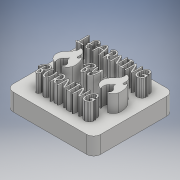
# Autodesk Inventor part: LearningByBurning
Saved by Autodesk Inventor 2017 (Build 210142000, 142)
## iProperties
Created: 2019-02-26
Part Number: LearningByBurning
Material: Generic
Document SubType Name: Modeling
Designer: Daniel Serena
Density: 1 g/cm^3
Appearance: Default
Author: Daniel Serena
Autodesk Inventor part; units mm, degrees
(part 1 of 2)
ref_plane "YZ Plane" through (0, 0, 0) normal (1, 0, 0) x (0, 1, 0)
ref_plane "XZ Plane" through (0, 0, 0) normal (0, 1, 0) x (-1, 0, 0)
ref_plane "XY Plane" through (0, 0, 0) normal (0, 0, 1) x (1, 0, 0)
sketch "Sketch1" plane through (0, 0, 0) normal (0, 0, 1) x (1, 0, 0)
  line L0 (-10.4772, 8.2772) -> (11.5644, 8.2772) construction
  line L1 (11.5644, 8.2772) -> (11.5644, -9.0375) construction
  line L2 (11.5644, -9.0375) -> (-10.4772, -9.0375) construction
  line L3 (-10.4772, -9.0375) -> (-10.4772, 8.2772) construction
  line L4 (-8.5891, 8.1961) -> (-8.5771, 8.1961)
  spline S0 degree 2 poles (-8.5771, 8.1961) (-8.4601, 8.1961) (-8.403, 8.0731) knots 0 0 0 1 1 1
  spline S1 degree 2 poles (-8.403, 8.0731) (-8.379, 8.0341) (-8.361, 7.6799) knots 0 0 0 1 1 1
  spline S2 degree 2 poles (-8.361, 7.6799) (-8.328, 7.0105) (-8.328, 6.3291) knots 0 0 0 1 1 1
  spline S3 degree 2 poles (-8.328, 6.3291) (-8.328, 5.4976) (-8.382, 5.0654) knots 0 0 0 1 1 1
  line L5 (-8.382, 5.0654) -> (-8.379, 5.0654)
  spline S4 degree 2 poles (-8.379, 5.0654) (-7.9408, 5.1764) (-7.6826, 5.1764) knots 0 0 0 1 1 1
  line L6 (-7.6826, 5.1764) -> (-7.6766, 5.1764)
  spline S5 degree 2 poles (-7.6766, 5.1764) (-7.3314, 5.1764) (-7.0733, 5.0143) knots 0 0 0 1 1 1
  spline S6 degree 2 poles (-7.0733, 5.0143) (-7.0072, 4.9483) (-7.0072, 4.8672) knots 0 0 0 1 1 1
  spline S7 degree 2 poles (-7.0072, 4.8672) (-7.0072, 4.7562) (-7.1183, 4.6931) knots 0 0 0 1 1 1
  spline S8 degree 2 poles (-7.1183, 4.6931) (-7.1603, 4.6721) (-7.2054, 4.6721) knots 0 0 0 1 1 1
  spline S9 degree 2 poles (-7.2054, 4.6721) (-7.2594, 4.6721) (-7.3704, 4.7352) knots 0 0 0 1 1 1
  spline S10 degree 2 poles (-7.3704, 4.7352) (-7.5175, 4.7862) (-7.6736, 4.7862) knots 0 0 0 1 1 1
  line L7 (-7.6736, 4.7862) -> (-7.6916, 4.7862)
  spline S11 degree 2 poles (-7.6916, 4.7862) (-7.9018, 4.7862) (-8.385, 4.6631) knots 0 0 0 1 1 1
  spline S12 degree 2 poles (-8.385, 4.6631) (-8.5921, 4.6181) (-8.7182, 4.6181) knots 0 0 0 1 1 1
  spline S13 degree 2 poles (-8.7182, 4.6181) (-9.0454, 4.6181) (-9.2135, 4.8913) knots 0 0 0 1 1 1
  spline S14 degree 2 poles (-9.2135, 4.8913) (-9.2345, 4.9333) (-9.2345, 4.9783) knots 0 0 0 1 1 1
  spline S15 degree 2 poles (-9.2345, 4.9783) (-9.2345, 5.0894) (-9.1204, 5.1524) knots 0 0 0 1 1 1
  spline S16 degree 2 poles (-9.1204, 5.1524) (-9.0934, 5.1674) (-9.0394, 5.1704) knots 0 0 0 1 1 1
  spline S17 degree 2 poles (-9.0394, 5.1704) (-8.9403, 5.1704) (-8.8683, 5.0684) knots 0 0 0 1 1 1
  spline S18 degree 2 poles (-8.8683, 5.0684) (-8.8263, 5.0323) (-8.7813, 5.0263) knots 0 0 0 1 1 1
  spline S19 degree 2 poles (-8.7813, 5.0263) (-8.7152, 5.3805) (-8.7152, 6.236) knots 0 0 0 1 1 1
  line L8 (-8.7152, 6.236) -> (-8.7152, 6.4672)
  spline S20 degree 2 poles (-8.7152, 6.4672) (-8.7152, 7.2776) (-8.7662, 7.929) knots 0 0 0 1 1 1
  spline S21 degree 2 poles (-8.7662, 7.929) (-8.7753, 7.974) (-8.7753, 8.004) knots 0 0 0 1 1 1
  spline S22 degree 2 poles (-8.7753, 8.004) (-8.7753, 8.1331) (-8.6312, 8.1901) knots 0 0 0 1 1 1
  spline S23 degree 2 poles (-8.6312, 8.1901) (-8.6012, 8.1961) (-8.5891, 8.1961) knots 0 0 0 1 1 1
  line L9 (-5.8096, 4.504) -> (-5.8426, 4.504)
  spline S24 degree 2 poles (-5.8426, 4.504) (-6.0677, 4.504) (-6.2598, 4.6661) knots 0 0 0 1 1 1
  spline S25 degree 2 poles (-6.2598, 4.6661) (-6.3859, 4.7922) (-6.4399, 4.9063) knots 0 0 0 1 1 1
  spline S26 degree 2 poles (-6.4399, 4.9063) (-6.4909, 5.0023) (-6.542, 5.1794) knots 0 0 0 1 1 1
  spline S27 degree 2 poles (-6.542, 5.1794) (-6.605, 5.4556) (-6.605, 5.5636) knots 0 0 0 1 1 1
  spline S28 degree 2 poles (-6.605, 5.5636) (-6.617, 5.6717) (-6.629, 5.8608) knots 0 0 0 1 1 1
  spline S29 degree 2 poles (-6.629, 5.8608) (-6.7491, 5.8008) (-6.8271, 5.8008) knots 0 0 0 1 1 1
  spline S30 degree 2 poles (-6.8271, 5.8008) (-6.9322, 5.8008) (-6.9622, 5.8998) knots 0 0 0 1 1 1
  spline S31 degree 2 poles (-6.9622, 5.8998) (-6.9682, 5.9268) (-6.9682, 5.9509) knots 0 0 0 1 1 1
  spline S32 degree 2 poles (-6.9682, 5.9509) (-6.9682, 6.122) (-6.647, 6.269) knots 0 0 0 1 1 1
  spline S33 degree 2 poles (-6.647, 6.269) (-6.644, 6.3681) (-6.644, 6.6503) knots 0 0 0 1 1 1
  spline S34 degree 2 poles (-6.644, 6.6503) (-6.644, 7.3617) (-6.563, 7.5958) knots 0 0 0 1 1 1
  spline S35 degree 2 poles (-6.563, 7.5958) (-6.4819, 7.875) (-6.3018, 8.0491) knots 0 0 0 1 1 1
  spline S36 degree 2 poles (-6.3018, 8.0491) (-6.0827, 8.2382) (-5.8036, 8.2382) knots 0 0 0 1 1 1
  spline S37 degree 2 poles (-5.8036, 8.2382) (-5.4554, 8.2382) (-5.1522, 7.977) knots 0 0 0 1 1 1
  spline S38 degree 2 poles (-5.1522, 7.977) (-4.906, 7.7459) (-4.906, 7.5028) knots 0 0 0 1 1 1
  spline S39 degree 2 poles (-4.906, 7.5028) (-4.906, 7.3707) (-4.9811, 7.2596) knots 0 0 0 1 1 1
  spline S40 degree 2 poles (-4.9811, 7.2596) (-5.0351, 7.1996) (-5.1132, 7.1996) knots 0 0 0 1 1 1
  spline S41 degree 2 poles (-5.1132, 7.1996) (-5.2302, 7.1996) (-5.2873, 7.3196) knots 0 0 0 1 1 1
  spline S42 degree 2 poles (-5.2873, 7.3196) (-5.2963, 7.3617) (-5.2963, 7.3767) knots 0 0 0 1 1 1
  spline S43 degree 2 poles (-5.2963, 7.3767) (-5.2963, 7.4097) (-5.2692, 7.4757) knots 0 0 0 1 1 1
  spline S44 degree 2 poles (-5.2692, 7.4757) (-5.2662, 7.4877) (-5.2662, 7.4967) knots 0 0 0 1 1 1
  spline S45 degree 2 poles (-5.2662, 7.4967) (-5.2662, 7.6378) (-5.4884, 7.7909) knots 0 0 0 1 1 1
  spline S46 degree 2 poles (-5.4884, 7.7909) (-5.6535, 7.884) (-5.8066, 7.884) knots 0 0 0 1 1 1
  spline S47 degree 2 poles (-5.8066, 7.884) (-6.1307, 7.884) (-6.2388, 7.4277) knots 0 0 0 1 1 1
  spline S48 degree 2 poles (-6.2388, 7.4277) (-6.2898, 7.2326) (-6.2898, 6.5362) knots 0 0 0 1 1 1
  line L10 (-6.2898, 6.5362) -> (-6.2868, 6.3561)
  spline S49 degree 2 poles (-6.2868, 6.3561) (-6.1127, 6.4011) (-5.9536, 6.4011) knots 0 0 0 1 1 1
  spline S50 degree 2 poles (-5.9536, 6.4011) (-5.7945, 6.4011) (-5.6355, 6.3591) knots 0 0 0 1 1 1
  spline S51 degree 2 poles (-5.6355, 6.3591) (-5.5304, 6.2961) (-5.5304, 6.209) knots 0 0 0 1 1 1
  line L11 (-5.5304, 6.209) -> (-5.5304, 6.179)
  spline S52 degree 2 poles (-5.5304, 6.179) (-5.5304, 6.107) (-5.6144, 6.0439) knots 0 0 0 1 1 1
  spline S53 degree 2 poles (-5.6144, 6.0439) (-5.6565, 6.0169) (-5.7075, 6.0169) knots 0 0 0 1 1 1
  spline S54 degree 2 poles (-5.7075, 6.0169) (-5.8966, 6.0439) (-5.9626, 6.0439) knots 0 0 0 1 1 1
  spline S55 degree 2 poles (-5.9626, 6.0439) (-6.1067, 6.0439) (-6.2748, 5.9839) knots 0 0 0 1 1 1
  spline S56 degree 2 poles (-6.2748, 5.9839) (-6.2748, 5.8218) (-6.2328, 5.4436) knots 0 0 0 1 1 1
  spline S57 degree 2 poles (-6.2328, 5.4436) (-6.1397, 4.8612) (-5.8246, 4.8612) knots 0 0 0 1 1 1
  spline S58 degree 2 poles (-5.8246, 4.8612) (-5.5964, 4.8612) (-5.2422, 5.1164) knots 0 0 0 1 1 1
  spline S59 degree 2 poles (-5.2422, 5.1164) (-5.1972, 5.1374) (-5.1612, 5.1374) knots 0 0 0 1 1 1
  spline S60 degree 2 poles (-5.1612, 5.1374) (-5.0411, 5.1374) (-4.9871, 5.0203) knots 0 0 0 1 1 1
  spline S61 degree 2 poles (-4.9871, 5.0203) (-4.9781, 4.9963) (-4.9781, 4.9633) knots 0 0 0 1 1 1
  spline S62 degree 2 poles (-4.9781, 4.9633) (-4.9781, 4.8492) (-5.1042, 4.7802) knots 0 0 0 1 1 1
  spline S63 degree 2 poles (-5.1042, 4.7802) (-5.5094, 4.504) (-5.8096, 4.504) knots 0 0 0 1 1 1
  spline S64 degree 2 poles (-3.3512, 8.2502) (-2.9159, 8.2502) (-2.6397, 7.4397) knots 0 0 0 1 1 1
  spline S65 degree 2 poles (-2.6397, 7.4397) (-2.5317, 7.1365) (-2.4296, 6.6413) knots 0 0 0 1 1 1
  spline S66 degree 2 poles (-2.4296, 6.6413) (-2.2345, 6.6232) (-2.2015, 6.5962) knots 0 0 0 1 1 1
  spline S67 degree 2 poles (-2.2015, 6.5962) (-2.1084, 6.5302) (-2.1084, 6.4251) knots 0 0 0 1 1 1
  spline S68 degree 2 poles (-2.1084, 6.4251) (-2.1084, 6.3171) (-2.2255, 6.248) knots 0 0 0 1 1 1
  spline S69 degree 2 poles (-2.2255, 6.248) (-2.2735, 6.236) (-2.3006, 6.236) knots 0 0 0 1 1 1
  spline S70 degree 2 poles (-2.3006, 6.236) (-2.3096, 6.236) (-2.3516, 6.239) knots 0 0 0 1 1 1
  spline S71 degree 2 poles (-2.3516, 6.239) (-2.1985, 5.2605) (-2.1234, 4.8913) knots 0 0 0 1 1 1
  spline S72 degree 2 poles (-2.1234, 4.8913) (-2.1174, 4.8913) (-2.1144, 4.8402) knots 0 0 0 1 1 1
  spline S73 degree 2 poles (-2.1144, 4.8402) (-2.1144, 4.7112) (-2.2555, 4.6541) knots 0 0 0 1 1 1
  spline S74 degree 2 poles (-2.2555, 4.6541) (-2.2915, 4.6481) (-2.3126, 4.6481) knots 0 0 0 1 1 1
  spline S75 degree 2 poles (-2.3126, 4.6481) (-2.4386, 4.6481) (-2.4957, 4.7862) knots 0 0 0 1 1 1
  spline S76 degree 2 poles (-2.4957, 4.7862) (-2.5797, 5.1884) (-2.7118, 6.0379) knots 0 0 0 1 1 1
  line L12 (-2.7118, 6.0379) -> (-2.7568, 6.2841)
  spline S77 degree 2 poles (-2.7568, 6.2841) (-3.2011, 6.3321) (-3.5913, 6.3321) knots 0 0 0 1 1 1
  spline S78 degree 2 poles (-3.5913, 6.3321) (-3.7984, 6.3321) (-3.9545, 6.3171) knots 0 0 0 1 1 1
  spline S79 degree 2 poles (-3.9545, 6.3171) (-4.0235, 5.8218) (-4.1166, 4.9033) knots 0 0 0 1 1 1
  spline S80 degree 2 poles (-4.1166, 4.9033) (-4.1466, 4.8102) (-4.2096, 4.7742) knots 0 0 0 1 1 1
  spline S81 degree 2 poles (-4.2096, 4.7742) (-4.2577, 4.7472) (-4.2997, 4.7472) knots 0 0 0 1 1 1
  line L13 (-4.2997, 4.7472) -> (-4.3237, 4.7472)
  spline S82 degree 2 poles (-4.3237, 4.7472) (-4.4288, 4.7472) (-4.4918, 4.8702) knots 0 0 0 1 1 1
  spline S83 degree 2 poles (-4.4918, 4.8702) (-4.5038, 4.9093) (-4.5038, 4.9423) knots 0 0 0 1 1 1
  spline S84 degree 2 poles (-4.5038, 4.9423) (-4.4078, 5.8728) (-4.3537, 6.248) knots 0 0 0 1 1 1
  line L14 (-4.3537, 6.248) -> (-4.3567, 6.248)
  spline S85 degree 2 poles (-4.3567, 6.248) (-4.4678, 6.218) (-4.5759, 6.158) knots 0 0 0 1 1 1
  spline S86 degree 2 poles (-4.5759, 6.158) (-4.6149, 6.128) (-4.6779, 6.128) knots 0 0 0 1 1 1
  spline S87 degree 2 poles (-4.6779, 6.128) (-4.81, 6.128) (-4.861, 6.257) knots 0 0 0 1 1 1
  spline S88 degree 2 poles (-4.861, 6.257) (-4.87, 6.2781) (-4.87, 6.3051) knots 0 0 0 1 1 1
  line L15 (-4.87, 6.3051) -> (-4.87, 6.3351)
  spline S89 degree 2 poles (-4.87, 6.3351) (-4.87, 6.4672) (-4.6629, 6.5452) knots 0 0 0 1 1 1
  spline S90 degree 2 poles (-4.6629, 6.5452) (-4.5969, 6.5842) (-4.3837, 6.6383) knots 0 0 0 1 1 1
  spline S91 degree 2 poles (-4.3837, 6.6383) (-4.2877, 6.6593) (-4.2847, 6.6653) knots 0 0 0 1 1 1
  spline S92 degree 2 poles (-4.2847, 6.6653) (-4.0085, 8.2502) (-3.3512, 8.2502) knots 0 0 0 1 1 1
  spline S93 degree 2 poles (-3.8885, 6.7073) (-3.7684, 6.7193) (-3.5673, 6.7193) knots 0 0 0 1 1 1
  line L16 (-3.5673, 6.7193) -> (-3.5493, 6.7193)
  spline S94 degree 2 poles (-3.5493, 6.7193) (-3.2071, 6.7193) (-2.8319, 6.6833) knots 0 0 0 1 1 1
  spline S95 degree 2 poles (-2.8319, 6.6833) (-3.066, 7.863) (-3.3481, 7.863) knots 0 0 0 1 1 1
  line L17 (-3.3481, 7.863) -> (-3.3632, 7.863)
  spline S96 degree 2 poles (-3.3632, 7.863) (-3.4652, 7.863) (-3.5733, 7.7159) knots 0 0 0 1 1 1
  spline S97 degree 2 poles (-3.5733, 7.7159) (-3.6453, 7.6078) (-3.7024, 7.4577) knots 0 0 0 1 1 1
  spline S98 degree 2 poles (-3.7024, 7.4577) (-3.7924, 7.2326) (-3.8885, 6.7073) knots 0 0 0 1 1 1
  line L18 (-1.0608, 4.474) -> (-1.0698, 4.474)
  spline S99 degree 2 poles (-1.0698, 4.474) (-1.265, 4.51) (-1.265, 4.6661) knots 0 0 0 1 1 1
  spline S100 degree 2 poles (-1.265, 4.6661) (-1.2169, 4.8492) (-1.2169, 5.4196) knots 0 0 0 1 1 1
  spline S101 degree 2 poles (-1.2169, 5.4196) (-1.2259, 5.6897) (-1.2259, 5.7618) knots 0 0 0 1 1 1
  spline S102 degree 2 poles (-1.2259, 5.7618) (-1.385, 5.7618) (-1.424, 5.9689) knots 0 0 0 1 1 1
  spline S103 degree 2 poles (-1.424, 5.9689) (-1.376, 6.164) (-1.2349, 6.164) knots 0 0 0 1 1 1
  line L19 (-1.2349, 6.164) -> (-1.265, 7.3587)
  spline S104 degree 2 poles (-1.265, 7.3587) (-1.265, 7.5808) (-1.0789, 7.5868) knots 0 0 0 1 1 1
  line L20 (-1.0789, 7.5868) -> (-1.0518, 7.5868)
  spline S105 degree 2 poles (-1.0518, 7.5868) (-0.8747, 7.5898) (-0.8657, 7.3887) knots 0 0 0 1 1 1
  spline S106 degree 2 poles (-0.8657, 7.3887) (-0.8747, 7.0975) (-0.8357, 6.134) knots 0 0 0 1 1 1
  spline S107 degree 2 poles (-0.8357, 6.134) (-0.3945, 6.134) (-0.1603, 6.5662) knots 0 0 0 1 1 1
  spline S108 degree 2 poles (-0.1603, 6.5662) (-0.0823, 6.7223) (-0.0823, 6.9054) knots 0 0 0 1 1 1
  line L21 (-0.0823, 6.9054) -> (-0.0823, 6.9955)
  spline S109 degree 2 poles (-0.0823, 6.9955) (-0.0823, 7.4187) (-0.3765, 7.7279) knots 0 0 0 1 1 1
  spline S110 degree 2 poles (-0.3765, 7.7279) (-0.5776, 7.884) (-0.8057, 7.884) knots 0 0 0 1 1 1
  spline S111 degree 2 poles (-0.8057, 7.884) (-1.1779, 7.884) (-1.346, 7.5718) knots 0 0 0 1 1 1
  spline S112 degree 2 poles (-1.346, 7.5718) (-1.4, 7.3677) (-1.5411, 7.3677) knots 0 0 0 1 1 1
  line L22 (-1.5411, 7.3677) -> (-1.5891, 7.3677)
  spline S113 degree 2 poles (-1.5891, 7.3677) (-1.7212, 7.3677) (-1.7542, 7.5628) knots 0 0 0 1 1 1
  spline S114 degree 2 poles (-1.7542, 7.5628) (-1.7542, 7.7789) (-1.4511, 8.0611) knots 0 0 0 1 1 1
  spline S115 degree 2 poles (-1.4511, 8.0611) (-1.1659, 8.2772) (-0.8057, 8.2772) knots 0 0 0 1 1 1
  spline S116 degree 2 poles (-0.8057, 8.2772) (-0.0012, 8.2772) (0.2719, 7.3467) knots 0 0 0 1 1 1
  spline S117 degree 2 poles (0.2719, 7.3467) (0.3199, 7.1035) (0.3199, 6.9354) knots 0 0 0 1 1 1
  spline S118 degree 2 poles (0.3199, 6.9354) (0.3199, 6.176) (-0.4035, 5.8218) knots 0 0 0 1 1 1
  spline S119 degree 2 poles (-0.4035, 5.8218) (-0.5415, 5.7828) (-0.5626, 5.7828) knots 0 0 0 1 1 1
  spline S120 degree 2 poles (-0.5626, 5.7828) (-0.3644, 5.4556) (-0.1423, 5.2154) knots 0 0 0 1 1 1
  spline S121 degree 2 poles (-0.1423, 5.2154) (-0.0463, 5.1194) (0.0138, 5.1074) knots 0 0 0 1 1 1
  spline S122 degree 2 poles (0.0138, 5.1074) (0.1188, 5.2365) (0.1909, 5.2365) knots 0 0 0 1 1 1
  line L23 (0.1909, 5.2365) -> (0.2299, 5.2365)
  spline S123 degree 2 poles (0.2299, 5.2365) (0.38, 5.2365) (0.416, 5.0383) knots 0 0 0 1 1 1
  spline S124 degree 2 poles (0.416, 5.0383) (0.416, 4.8582) (0.1038, 4.7262) knots 0 0 0 1 1 1
  spline S125 degree 2 poles (0.1038, 4.7262) (0.0648, 4.7172) (0.0228, 4.7172) knots 0 0 0 1 1 1
  spline S126 degree 2 poles (0.0228, 4.7172) (-0.3524, 4.7172) (-0.7967, 5.4196) knots 0 0 0 1 1 1
  line L24 (-0.7967, 5.4196) -> (-0.8267, 5.4496)
  line L25 (-0.8267, 5.4496) -> (-0.8267, 5.2845)
  spline S127 degree 2 poles (-0.8267, 5.2845) (-0.8267, 4.5401) (-0.9228, 4.5401) knots 0 0 0 1 1 1
  spline S128 degree 2 poles (-0.9228, 4.5401) (-0.9228, 4.498) (-1.0608, 4.474) knots 0 0 0 1 1 1
  line L26 (2.5292, 8.1121) -> (2.5622, 8.1121)
  spline S129 degree 2 poles (2.5622, 8.1121) (2.6403, 8.1121) (2.7123, 8.019) knots 0 0 0 1 1 1
  spline S130 degree 2 poles (2.7123, 8.019) (2.7453, 7.977) (2.7453, 7.7879) knots 0 0 0 1 1 1
  spline S131 degree 2 poles (2.7453, 7.7879) (2.7693, 7.1305) (2.7693, 6.5782) knots 0 0 0 1 1 1
  line L27 (2.7693, 6.5782) -> (2.7693, 6.5512)
  spline S132 degree 2 poles (2.7693, 6.5512) (2.7693, 5.2965) (2.6013, 4.9813) knots 0 0 0 1 1 1
  spline S133 degree 2 poles (2.6013, 4.9813) (2.5352, 4.8642) (2.4392, 4.8642) knots 0 0 0 1 1 1
  spline S134 degree 2 poles (2.4392, 4.8642) (2.232, 4.8642) (2.0129, 5.3475) knots 0 0 0 1 1 1
  spline S135 degree 2 poles (2.0129, 5.3475) (1.8988, 5.5967) (1.6167, 6.2871) knots 0 0 0 1 1 1
  spline S136 degree 2 poles (1.6167, 6.2871) (1.3705, 6.8574) (1.1394, 7.2176) knots 0 0 0 1 1 1
  line L28 (1.1394, 7.2176) -> (1.1364, 7.2176)
  spline S137 degree 2 poles (1.1364, 7.2176) (1.1364, 7.1696) (1.1334, 6.9955) knots 0 0 0 1 1 1
  line L29 (1.1334, 6.9955) -> (1.1424, 5.8068)
  spline S138 degree 2 poles (1.1424, 5.8068) (1.1424, 4.7502) (0.9953, 4.6631) knots 0 0 0 1 1 1
  spline S139 degree 2 poles (0.9953, 4.6631) (0.9413, 4.6151) (0.8813, 4.6151) knots 0 0 0 1 1 1
  line L30 (0.8813, 4.6151) -> (0.8723, 4.6151)
  spline S140 degree 2 poles (0.8723, 4.6151) (0.7402, 4.6151) (0.6862, 4.7562) knots 0 0 0 1 1 1
  spline S141 degree 2 poles (0.6862, 4.7562) (0.6772, 4.7892) (0.6772, 4.8102) knots 0 0 0 1 1 1
  spline S142 degree 2 poles (0.6772, 4.8102) (0.6772, 4.8312) (0.7102, 4.9663) knots 0 0 0 1 1 1
  spline S143 degree 2 poles (0.7102, 4.9663) (0.7552, 5.2094) (0.7552, 5.7377) knots 0 0 0 1 1 1
  line L31 (0.7552, 5.7377) -> (0.7552, 5.8188)
  spline S144 degree 2 poles (0.7552, 5.8188) (0.7552, 6.0409) (0.7462, 6.7523) knots 0 0 0 1 1 1
  spline S145 degree 2 poles (0.7462, 6.7523) (0.7462, 7.5958) (0.8843, 7.7249) knots 0 0 0 1 1 1
  spline S146 degree 2 poles (0.8843, 7.7249) (0.9743, 7.8089) (1.0524, 7.8089) knots 0 0 0 1 1 1
  spline S147 degree 2 poles (1.0524, 7.8089) (1.1934, 7.8089) (1.3766, 7.5538) knots 0 0 0 1 1 1
  spline S148 degree 2 poles (1.3766, 7.5538) (1.5567, 7.3076) (1.7338, 6.9564) knots 0 0 0 1 1 1
  spline S149 degree 2 poles (1.7338, 6.9564) (1.9709, 6.4702) (2.3161, 5.6147) knots 0 0 0 1 1 1
  spline S150 degree 2 poles (2.3161, 5.6147) (2.3671, 5.4946) (2.3911, 5.4736) knots 0 0 0 1 1 1
  line L32 (2.3911, 5.4736) -> (2.4001, 5.4736)
  spline S151 degree 2 poles (2.4001, 5.4736) (2.4091, 5.5907) (2.4091, 5.7588) knots 0 0 0 1 1 1
  spline S152 degree 2 poles (2.4091, 5.7588) (2.4091, 6.3651) (2.3521, 7.923) knots 0 0 0 1 1 1
  spline S153 degree 2 poles (2.3521, 7.923) (2.3521, 8.022) (2.4602, 8.0911) knots 0 0 0 1 1 1
  spline S154 degree 2 poles (2.4602, 8.0911) (2.5052, 8.1121) (2.5292, 8.1121) knots 0 0 0 1 1 1
  line L33 (3.7809, 8.2202) -> (3.8079, 8.2202)
  spline S155 degree 2 poles (3.8079, 8.2202) (3.907, 8.2202) (3.973, 8.1061) knots 0 0 0 1 1 1
  spline S156 degree 2 poles (3.973, 8.1061) (3.982, 8.0791) (3.982, 8.0761) knots 0 0 0 1 1 1
  spline S157 degree 2 poles (3.982, 8.0761) (4.2612, 8.0851) (4.2612, 8.1031) knots 0 0 0 1 1 1
  spline S158 degree 2 poles (4.2612, 8.1031) (4.2972, 8.1151) (4.3302, 8.1151) knots 0 0 0 1 1 1
  spline S159 degree 2 poles (4.3302, 8.1151) (4.4683, 8.1151) (4.5163, 7.971) knots 0 0 0 1 1 1
  spline S160 degree 2 poles (4.5163, 7.971) (4.5223, 7.953) (4.5253, 7.92) knots 0 0 0 1 1 1
  spline S161 degree 2 poles (4.5253, 7.92) (4.5253, 7.8119) (4.4143, 7.7459) knots 0 0 0 1 1 1
  spline S162 degree 2 poles (4.4143, 7.7459) (4.3392, 7.7279) (4.0661, 7.7039) knots 0 0 0 1 1 1
  spline S163 degree 2 poles (4.0661, 7.7039) (4.1231, 7.3166) (4.1231, 6.6353) knots 0 0 0 1 1 1
  spline S164 degree 2 poles (4.1231, 6.6353) (4.1231, 6.3561) (4.1021, 5.1914) knots 0 0 0 1 1 1
  line L34 (4.1021, 5.1914) -> (4.1021, 5.1464)
  spline S165 degree 2 poles (4.1021, 5.1464) (4.3783, 5.1584) (4.4113, 5.1674) knots 0 0 0 1 1 1
  spline S166 degree 2 poles (4.4113, 5.1674) (4.5344, 5.1674) (4.5944, 5.0353) knots 0 0 0 1 1 1
  spline S167 degree 2 poles (4.5944, 5.0353) (4.6064, 4.9993) (4.6064, 4.9723) knots 0 0 0 1 1 1
  line L35 (4.6064, 4.9723) -> (4.6064, 4.9693)
  spline S168 degree 2 poles (4.6064, 4.9693) (4.6064, 4.8372) (4.4623, 4.7802) knots 0 0 0 1 1 1
  spline S169 degree 2 poles (4.4623, 4.7802) (4.3482, 4.7682) (3.4297, 4.7292) knots 0 0 0 1 1 1
  spline S170 degree 2 poles (3.4297, 4.7292) (3.3217, 4.7292) (3.2586, 4.8402) knots 0 0 0 1 1 1
  spline S171 degree 2 poles (3.2586, 4.8402) (3.2406, 4.8793) (3.2406, 4.9213) knots 0 0 0 1 1 1
  line L36 (3.2406, 4.9213) -> (3.2406, 4.9303)
  spline S172 degree 2 poles (3.2406, 4.9303) (3.2406, 5.0353) (3.3517, 5.0984) knots 0 0 0 1 1 1
  spline S173 degree 2 poles (3.3517, 5.0984) (3.3847, 5.1224) (3.5768, 5.1224) knots 0 0 0 1 1 1
  spline S174 degree 2 poles (3.5768, 5.1224) (3.5768, 5.1254) (3.7089, 5.1284) knots 0 0 0 1 1 1
  spline S175 degree 2 poles (3.7089, 5.1284) (3.7359, 6.266) (3.7359, 6.5452) knots 0 0 0 1 1 1
  line L37 (3.7359, 6.5452) -> (3.7359, 6.7283)
  spline S176 degree 2 poles (3.7359, 6.7283) (3.7359, 7.3226) (3.6759, 7.6768) knots 0 0 0 1 1 1
  spline S177 degree 2 poles (3.6759, 7.6768) (3.6579, 7.6768) (3.2676, 7.6468) knots 0 0 0 1 1 1
  spline S178 degree 2 poles (3.2676, 7.6468) (3.1776, 7.6468) (3.1085, 7.7339) knots 0 0 0 1 1 1
  spline S179 degree 2 poles (3.1085, 7.7339) (3.0785, 7.7849) (3.0785, 7.8329) knots 0 0 0 1 1 1
  line L38 (3.0785, 7.8329) -> (3.0785, 7.8509)
  spline S180 degree 2 poles (3.0785, 7.8509) (3.0785, 7.95) (3.1836, 8.013) knots 0 0 0 1 1 1
  spline S181 degree 2 poles (3.1836, 8.013) (3.2286, 8.0371) (3.2946, 8.0401) knots 0 0 0 1 1 1
  spline S182 degree 2 poles (3.2946, 8.0401) (3.5858, 8.0581) (3.6068, 8.0611) knots 0 0 0 1 1 1
  spline S183 degree 2 poles (3.6068, 8.0611) (3.6068, 8.1121) (3.6759, 8.1811) knots 0 0 0 1 1 1
  spline S184 degree 2 poles (3.6759, 8.1811) (3.7389, 8.2202) (3.7809, 8.2202) knots 0 0 0 1 1 1
  line L39 (6.8727, 8.1121) -> (6.9057, 8.1121)
  spline S185 degree 2 poles (6.9057, 8.1121) (6.9838, 8.1121) (7.0558, 8.019) knots 0 0 0 1 1 1
  spline S186 degree 2 poles (7.0558, 8.019) (7.0888, 7.977) (7.0888, 7.7879) knots 0 0 0 1 1 1
  spline S187 degree 2 poles (7.0888, 7.7879) (7.1128, 7.1305) (7.1128, 6.5782) knots 0 0 0 1 1 1
  line L40 (7.1128, 6.5782) -> (7.1128, 6.5512)
  spline S188 degree 2 poles (7.1128, 6.5512) (7.1128, 5.2965) (6.9447, 4.9813) knots 0 0 0 1 1 1
  spline S189 degree 2 poles (6.9447, 4.9813) (6.8787, 4.8642) (6.7826, 4.8642) knots 0 0 0 1 1 1
  spline S190 degree 2 poles (6.7826, 4.8642) (6.5755, 4.8642) (6.3564, 5.3475) knots 0 0 0 1 1 1
  spline S191 degree 2 poles (6.3564, 5.3475) (6.2423, 5.5967) (5.9602, 6.2871) knots 0 0 0 1 1 1
  spline S192 degree 2 poles (5.9602, 6.2871) (5.714, 6.8574) (5.4829, 7.2176) knots 0 0 0 1 1 1
  line L41 (5.4829, 7.2176) -> (5.4799, 7.2176)
  spline S193 degree 2 poles (5.4799, 7.2176) (5.4799, 7.1696) (5.4769, 6.9955) knots 0 0 0 1 1 1
  line L42 (5.4769, 6.9955) -> (5.4859, 5.8068)
  spline S194 degree 2 poles (5.4859, 5.8068) (5.4859, 4.7502) (5.3388, 4.6631) knots 0 0 0 1 1 1
  spline S195 degree 2 poles (5.3388, 4.6631) (5.2848, 4.6151) (5.2247, 4.6151) knots 0 0 0 1 1 1
  line L43 (5.2247, 4.6151) -> (5.2157, 4.6151)
  spline S196 degree 2 poles (5.2157, 4.6151) (5.0837, 4.6151) (5.0296, 4.7562) knots 0 0 0 1 1 1
  spline S197 degree 2 poles (5.0296, 4.7562) (5.0206, 4.7892) (5.0206, 4.8102) knots 0 0 0 1 1 1
  spline S198 degree 2 poles (5.0206, 4.8102) (5.0206, 4.8312) (5.0537, 4.9663) knots 0 0 0 1 1 1
  spline S199 degree 2 poles (5.0537, 4.9663) (5.0987, 5.2094) (5.0987, 5.7377) knots 0 0 0 1 1 1
  line L44 (5.0987, 5.7377) -> (5.0987, 5.8188)
  spline S200 degree 2 poles (5.0987, 5.8188) (5.0987, 6.0409) (5.0897, 6.7523) knots 0 0 0 1 1 1
  spline S201 degree 2 poles (5.0897, 6.7523) (5.0897, 7.5958) (5.2278, 7.7249) knots 0 0 0 1 1 1
  spline S202 degree 2 poles (5.2278, 7.7249) (5.3178, 7.8089) (5.3958, 7.8089) knots 0 0 0 1 1 1
  spline S203 degree 2 poles (5.3958, 7.8089) (5.5369, 7.8089) (5.72, 7.5538) knots 0 0 0 1 1 1
  spline S204 degree 2 poles (5.72, 7.5538) (5.9001, 7.3076) (6.0772, 6.9564) knots 0 0 0 1 1 1
  spline S205 degree 2 poles (6.0772, 6.9564) (6.3144, 6.4702) (6.6596, 5.6147) knots 0 0 0 1 1 1
  spline S206 degree 2 poles (6.6596, 5.6147) (6.7106, 5.4946) (6.7346, 5.4736) knots 0 0 0 1 1 1
  line L45 (6.7346, 5.4736) -> (6.7436, 5.4736)
  spline S207 degree 2 poles (6.7436, 5.4736) (6.7526, 5.5907) (6.7526, 5.7588) knots 0 0 0 1 1 1
  spline S208 degree 2 poles (6.7526, 5.7588) (6.7526, 6.3651) (6.6956, 7.923) knots 0 0 0 1 1 1
  spline S209 degree 2 poles (6.6956, 7.923) (6.6956, 8.022) (6.8037, 8.0911) knots 0 0 0 1 1 1
  spline S210 degree 2 poles (6.8037, 8.0911) (6.8487, 8.1121) (6.8727, 8.1121) knots 0 0 0 1 1 1
  line L46 (8.8418, 8.2112) -> (8.8538, 8.2112)
  spline S211 degree 2 poles (8.8538, 8.2112) (9.205, 8.2112) (9.4932, 7.959) knots 0 0 0 1 1 1
  spline S212 degree 2 poles (9.4932, 7.959) (9.6313, 7.8239) (9.6853, 7.7279) knots 0 0 0 1 1 1
  spline S213 degree 2 poles (9.6853, 7.7279) (9.8384, 7.4577) (9.8384, 7.1606) knots 0 0 0 1 1 1
  spline S214 degree 2 poles (9.8384, 7.1606) (9.8384, 7.0525) (9.7333, 6.9895) knots 0 0 0 1 1 1
  spline S215 degree 2 poles (9.7333, 6.9895) (9.6883, 6.9684) (9.6433, 6.9684) knots 0 0 0 1 1 1
  spline S216 degree 2 poles (9.6433, 6.9684) (9.5172, 6.9684) (9.4632, 7.0975) knots 0 0 0 1 1 1
  spline S217 degree 2 poles (9.4632, 7.0975) (9.4542, 7.0975) (9.4422, 7.2746) knots 0 0 0 1 1 1
  spline S218 degree 2 poles (9.4422, 7.2746) (9.4151, 7.4067) (9.3791, 7.4757) knots 0 0 0 1 1 1
  spline S219 degree 2 poles (9.3791, 7.4757) (9.3461, 7.5538) (9.238, 7.6648) knots 0 0 0 1 1 1
  spline S220 degree 2 poles (9.238, 7.6648) (9.0549, 7.8209) (8.8598, 7.8209) knots 0 0 0 1 1 1
  line L47 (8.8598, 7.8209) -> (8.8388, 7.8209)
  spline S221 degree 2 poles (8.8388, 7.8209) (8.5537, 7.8209) (8.3045, 7.5058) knots 0 0 0 1 1 1
  spline S222 degree 2 poles (8.3045, 7.5058) (8.2055, 7.3587) (8.1544, 7.2386) knots 0 0 0 1 1 1
  spline S223 degree 2 poles (8.1544, 7.2386) (8.0734, 7.0555) (8.0043, 6.7223) knots 0 0 0 1 1 1
  spline S224 degree 2 poles (8.0043, 6.7223) (7.9503, 6.3831) (7.9503, 6.11) knots 0 0 0 1 1 1
  line L48 (7.9503, 6.11) -> (7.9503, 6.0769)
  spline S225 degree 2 poles (7.9503, 6.0769) (7.9503, 5.4346) (8.2535, 5.1674) knots 0 0 0 1 1 1
  spline S226 degree 2 poles (8.2535, 5.1674) (8.4246, 5.0233) (8.6707, 5.0233) knots 0 0 0 1 1 1
  spline S227 degree 2 poles (8.6707, 5.0233) (9.0549, 5.0233) (9.4512, 5.3205) knots 0 0 0 1 1 1
  spline S228 degree 2 poles (9.4512, 5.3205) (9.6643, 5.4946) (9.7183, 5.6927) knots 0 0 0 1 1 1
  spline S229 degree 2 poles (9.7183, 5.6927) (9.7243, 5.7317) (9.7243, 5.7437) knots 0 0 0 1 1 1
  spline S230 degree 2 poles (9.7243, 5.7437) (9.7243, 5.9779) (9.2711, 6.11) knots 0 0 0 1 1 1
  spline S231 degree 2 poles (9.2711, 6.11) (9.127, 6.0589) (9.127, 5.9989) knots 0 0 0 1 1 1
  spline S232 degree 2 poles (9.127, 5.9989) (9.088, 5.9208) (9.0069, 5.8908) knots 0 0 0 1 1 1
  spline S233 degree 2 poles (9.0069, 5.8908) (8.9709, 5.8818) (8.9589, 5.8818) knots 0 0 0 1 1 1
  line L49 (8.9589, 5.8818) -> (8.9319, 5.8818)
  spline S234 degree 2 poles (8.9319, 5.8818) (8.8358, 5.8818) (8.7728, 5.9899) knots 0 0 0 1 1 1
  spline S235 degree 2 poles (8.7728, 5.9899) (8.7518, 6.0379) (8.7518, 6.0799) knots 0 0 0 1 1 1
  spline S236 degree 2 poles (8.7518, 6.0799) (8.7518, 6.188) (8.8898, 6.3321) knots 0 0 0 1 1 1
  spline S237 degree 2 poles (8.8898, 6.3321) (9.0399, 6.4612) (9.2861, 6.5242) knots 0 0 0 1 1 1
  spline S238 degree 2 poles (9.2861, 6.5242) (9.5382, 6.5782) (9.7934, 6.5782) knots 0 0 0 1 1 1
  line L50 (9.7934, 6.5782) -> (9.8414, 6.5782)
  spline S239 degree 2 poles (9.8414, 6.5782) (10.0185, 6.5782) (10.0515, 6.5542) knots 0 0 0 1 1 1
  spline S240 degree 2 poles (10.0515, 6.5542) (10.1536, 6.4852) (10.1536, 6.3771) knots 0 0 0 1 1 1
  spline S241 degree 2 poles (10.1536, 6.3771) (10.1536, 6.26) (10.0305, 6.197) knots 0 0 0 1 1 1
  spline S242 degree 2 poles (10.0305, 6.197) (10.0155, 6.191) (9.9615, 6.185) knots 0 0 0 1 1 1
  line L51 (9.9615, 6.185) -> (9.9464, 6.188)
  line L52 (9.9464, 6.188) -> (9.9404, 6.188)
  spline S243 degree 2 poles (9.9404, 6.188) (10.1145, 5.9989) (10.1145, 5.7828) knots 0 0 0 1 1 1
  line L53 (10.1145, 5.7828) -> (10.1145, 5.7467)
  spline S244 degree 2 poles (10.1145, 5.7467) (10.1145, 5.5066) (9.9134, 5.2455) knots 0 0 0 1 1 1
  spline S245 degree 2 poles (9.9134, 5.2455) (9.7543, 5.0564) (9.6493, 4.9843) knots 0 0 0 1 1 1
  spline S246 degree 2 poles (9.6493, 4.9843) (9.4782, 4.8582) (9.3191, 4.7862) knots 0 0 0 1 1 1
  spline S247 degree 2 poles (9.3191, 4.7862) (8.9769, 4.6361) (8.7037, 4.6361) knots 0 0 0 1 1 1
  line L54 (8.7037, 4.6361) -> (8.6317, 4.6361)
  spline S248 degree 2 poles (8.6317, 4.6361) (8.3645, 4.6361) (8.1064, 4.7832) knots 0 0 0 1 1 1
  spline S249 degree 2 poles (8.1064, 4.7832) (7.8212, 4.9513) (7.6772, 5.3355) knots 0 0 0 1 1 1
  spline S250 degree 2 poles (7.6772, 5.3355) (7.5601, 5.6537) (7.5601, 6.0499) knots 0 0 0 1 1 1
  line L55 (7.5601, 6.0499) -> (7.5601, 6.131)
  spline S251 degree 2 poles (7.5601, 6.131) (7.5601, 6.5662) (7.6802, 7.0555) knots 0 0 0 1 1 1
  spline S252 degree 2 poles (7.6802, 7.0555) (7.7702, 7.3497) (7.8693, 7.5328) knots 0 0 0 1 1 1
  spline S253 degree 2 poles (7.8693, 7.5328) (7.9443, 7.6859) (8.0914, 7.8509) knots 0 0 0 1 1 1
  spline S254 degree 2 poles (8.0914, 7.8509) (8.2265, 7.995) (8.3075, 8.0431) knots 0 0 0 1 1 1
  spline S255 degree 2 poles (8.3075, 8.0431) (8.5657, 8.2112) (8.8418, 8.2112) knots 0 0 0 1 1 1
  spline S256 degree 2 poles (-0.5355, 1.8306) (-0.1663, 1.8306) (0.1038, 1.5845) knots 0 0 0 1 1 1
  spline S257 degree 2 poles (0.1038, 1.5845) (0.365, 1.3173) (0.365, 0.9421) knots 0 0 0 1 1 1
  spline S258 degree 2 poles (0.365, 0.9421) (0.365, 0.4228) (-0.1483, -0.1205) knots 0 0 0 1 1 1
  spline S259 degree 2 poles (-0.1483, -0.1205) (-0.3134, -0.2826) (-0.4365, -0.3817) knots 0 0 0 1 1 1
  spline S260 degree 2 poles (-0.4365, -0.3817) (-0.1393, -0.5618) (-0.0192, -0.901) knots 0 0 0 1 1 1
  spline S261 degree 2 poles (-0.0192, -0.901) (0.0378, -1.0691) (0.0378, -1.2462) knots 0 0 0 1 1 1
  line L56 (0.0378, -1.2462) -> (0.0378, -1.2582)
  spline S262 degree 2 poles (0.0378, -1.2582) (0.0378, -1.5914) (-0.1603, -1.8855) knots 0 0 0 1 1 1
  spline S263 degree 2 poles (-0.1603, -1.8855) (-0.3734, -2.1647) (-0.6466, -2.1647) knots 0 0 0 1 1 1
  spline S264 degree 2 poles (-0.6466, -2.1647) (-1.1809, -2.1647) (-1.286, -1.1861) knots 0 0 0 1 1 1
  spline S265 degree 2 poles (-1.286, -1.1861) (-1.31, -0.961) (-1.31, -0.6968) knots 0 0 0 1 1 1
  spline S266 degree 2 poles (-1.31, -0.6968) (-1.31, -0.0845) (-1.1959, 0.801) knots 0 0 0 1 1 1
  spline S267 degree 2 poles (-1.1959, 0.801) (-1.1779, 0.8701) (-1.1119, 0.9211) knots 0 0 0 1 1 1
  spline S268 degree 2 poles (-1.1119, 0.9211) (-1.0518, 0.9481) (-1.0038, 0.9481) knots 0 0 0 1 1 1
  spline S269 degree 2 poles (-1.0038, 0.9481) (-0.8927, 0.9481) (-0.8297, 0.837) knots 0 0 0 1 1 1
  spline S270 degree 2 poles (-0.8297, 0.837) (-0.8147, 0.798) (-0.8147, 0.756) knots 0 0 0 1 1 1
  line L57 (-0.8147, 0.756) -> (-0.8147, 0.753)
  spline S271 degree 2 poles (-0.8147, 0.753) (-0.8717, 0.2967) (-0.9078, -0.2436) knots 0 0 0 1 1 1
  spline S272 degree 2 poles (-0.9078, -0.2436) (-0.7577, -0.1475) (-0.5235, 0.0566) knots 0 0 0 1 1 1
  spline S273 degree 2 poles (-0.5235, 0.0566) (-0.0222, 0.5279) (-0.0222, 0.9391) knots 0 0 0 1 1 1
  line L58 (-0.0222, 0.9391) -> (-0.0222, 0.9451)
  spline S274 degree 2 poles (-0.0222, 0.9451) (-0.0222, 1.2273) (-0.2594, 1.3713) knots 0 0 0 1 1 1
  spline S275 degree 2 poles (-0.2594, 1.3713) (-0.3885, 1.4434) (-0.5085, 1.4434) knots 0 0 0 1 1 1
  line L59 (-0.5085, 1.4434) -> (-0.5656, 1.4434)
  spline S276 degree 2 poles (-0.5656, 1.4434) (-0.7637, 1.4434) (-1.0128, 1.2843) knots 0 0 0 1 1 1
  spline S277 degree 2 poles (-1.0128, 1.2843) (-1.0909, 1.2303) (-1.1749, 1.1492) knots 0 0 0 1 1 1
  spline S278 degree 2 poles (-1.1749, 1.1492) (-1.34, 0.9871) (-1.388, 0.9091) knots 0 0 0 1 1 1
  spline S279 degree 2 poles (-1.388, 0.9091) (-1.5711, 0.6419) (-1.6762, 0.3688) knots 0 0 0 1 1 1
  spline S280 degree 2 poles (-1.6762, 0.3688) (-1.7422, 0.2157) (-1.8113, -0.0215) knots 0 0 0 1 1 1
  spline S281 degree 2 poles (-1.8113, -0.0215) (-1.8713, -0.1385) (-1.9944, -0.1385) knots 0 0 0 1 1 1
  spline S282 degree 2 poles (-1.9944, -0.1385) (-2.1024, -0.1385) (-2.1655, -0.0245) knots 0 0 0 1 1 1
  spline S283 degree 2 poles (-2.1655, -0.0245) (-2.1835, 0.0116) (-2.1835, 0.0566) knots 0 0 0 1 1 1
  spline S284 degree 2 poles (-2.1835, 0.0566) (-2.1715, 0.2067) (-1.9614, 0.69) knots 0 0 0 1 1 1
  spline S285 degree 2 poles (-1.9614, 0.69) (-1.8473, 0.9301) (-1.6612, 1.1882) knots 0 0 0 1 1 1
  spline S286 degree 2 poles (-1.6612, 1.1882) (-1.5951, 1.2843) (-1.397, 1.4734) knots 0 0 0 1 1 1
  spline S287 degree 2 poles (-1.397, 1.4734) (-0.9858, 1.8306) (-0.5355, 1.8306) knots 0 0 0 1 1 1
  line L60 (-0.9198, -0.5948) -> (-0.9198, -0.7179)
  spline S288 degree 2 poles (-0.9198, -0.7179) (-0.9198, -1.3392) (-0.7907, -1.6604) knots 0 0 0 1 1 1
  spline S289 degree 2 poles (-0.7907, -1.6604) (-0.7277, -1.7745) (-0.6676, -1.7745) knots 0 0 0 1 1 1
  line L61 (-0.6676, -1.7745) -> (-0.6436, -1.7745)
  spline S290 degree 2 poles (-0.6436, -1.7745) (-0.5265, -1.7745) (-0.4065, -1.5463) knots 0 0 0 1 1 1
  spline S291 degree 2 poles (-0.4065, -1.5463) (-0.3464, -1.3932) (-0.3464, -1.2492) knots 0 0 0 1 1 1
  spline S292 degree 2 poles (-0.3464, -1.2492) (-0.3464, -0.8799) (-0.6946, -0.6848) knots 0 0 0 1 1 1
  spline S293 degree 2 poles (-0.6946, -0.6848) (-0.7907, -0.6368) (-0.9138, -0.5978) knots 0 0 0 1 1 1
  spline S294 degree 2 poles (-0.9138, -0.5978) (-0.9138, -0.5978) (-0.9198, -0.5948) knots 0 0 0 1 1 1
  spline S295 degree 2 poles (1.9979, 1.5394) (2.097, 1.5394) (2.163, 1.4464) knots 0 0 0 1 1 1
  spline S296 degree 2 poles (2.163, 1.4464) (2.3251, 1.0952) (2.3251, 0.4528) knots 0 0 0 1 1 1
  line L62 (2.3251, 0.4528) -> (2.3251, 0.4408)
  spline S297 degree 2 poles (2.3251, 0.4408) (2.3251, -0.3877) (2.0699, -1.2311) knots 0 0 0 1 1 1
  spline S298 degree 2 poles (2.0699, -1.2311) (1.7758, -2.1317) (1.2745, -2.1317) knots 0 0 0 1 1 1
  spline S299 degree 2 poles (1.2745, -2.1317) (1.0133, -2.1317) (0.7972, -1.8615) knots 0 0 0 1 1 1
  spline S300 degree 2 poles (0.7972, -1.8615) (0.7192, -1.7534) (0.6802, -1.6484) knots 0 0 0 1 1 1
  spline S301 degree 2 poles (0.6802, -1.6484) (0.6051, -1.4533) (0.6051, -1.3002) knots 0 0 0 1 1 1
  line L63 (0.6051, -1.3002) -> (0.6051, -1.2311)
  spline S302 degree 2 poles (0.6051, -1.2311) (0.6051, -1.0841) (0.6651, -0.952) knots 0 0 0 1 1 1
  spline S303 degree 2 poles (0.6651, -0.952) (0.7342, -0.8559) (0.8332, -0.8559) knots 0 0 0 1 1 1
  spline S304 degree 2 poles (0.8332, -0.8559) (0.9473, -0.8559) (1.0103, -0.973) knots 0 0 0 1 1 1
  spline S305 degree 2 poles (1.0103, -0.973) (1.0253, -1.012) (1.0253, -1.054) knots 0 0 0 1 1 1
  spline S306 degree 2 poles (1.0253, -1.054) (1.0253, -1.0721) (0.9953, -1.2011) knots 0 0 0 1 1 1
  spline S307 degree 2 poles (0.9953, -1.2011) (0.9923, -1.2401) (0.9923, -1.2582) knots 0 0 0 1 1 1
  line L64 (0.9923, -1.2582) -> (0.9923, -1.2762)
  spline S308 degree 2 poles (0.9923, -1.2762) (0.9923, -1.4893) (1.1394, -1.6664) knots 0 0 0 1 1 1
  spline S309 degree 2 poles (1.1394, -1.6664) (1.2115, -1.7444) (1.2805, -1.7444) knots 0 0 0 1 1 1
  spline S310 degree 2 poles (1.2805, -1.7444) (1.4366, -1.7444) (1.6107, -1.3512) knots 0 0 0 1 1 1
  spline S311 degree 2 poles (1.6107, -1.3512) (1.7007, -1.1561) (1.8058, -0.7209) knots 0 0 0 1 1 1
  spline S312 degree 2 poles (1.8058, -0.7209) (1.9379, -0.0875) (1.9379, 0.4618) knots 0 0 0 1 1 1
  spline S313 degree 2 poles (1.9379, 0.4618) (1.9349, 0.4858) (1.9349, 0.5309) knots 0 0 0 1 1 1
  line L65 (1.9349, 0.5309) -> (1.9349, 0.5819)
  line L66 (1.9349, 0.5819) -> (1.9349, 0.6089)
  line L67 (1.9349, 0.6089) -> (1.9319, 0.6089)
  spline S314 degree 2 poles (1.9319, 0.6089) (1.4696, -0.6158) (1.0824, -0.6158) knots 0 0 0 1 1 1
  spline S315 degree 2 poles (1.0824, -0.6158) (0.5661, -0.6158) (0.458, 1.2933) knots 0 0 0 1 1 1
  line L68 (0.458, 1.2933) -> (0.458, 1.3233)
  spline S316 degree 2 poles (0.458, 1.3233) (0.458, 1.4314) (0.5751, 1.4944) knots 0 0 0 1 1 1
  spline S317 degree 2 poles (0.5751, 1.4944) (0.6171, 1.5094) (0.6561, 1.5094) knots 0 0 0 1 1 1
  spline S318 degree 2 poles (0.6561, 1.5094) (0.7792, 1.5094) (0.8332, 1.3803) knots 0 0 0 1 1 1
  spline S319 degree 2 poles (0.8332, 1.3803) (0.8482, 1.3803) (0.8633, 1.0291) knots 0 0 0 1 1 1
  spline S320 degree 2 poles (0.8633, 1.0291) (0.9443, -0.2256) (1.0734, -0.2256) knots 0 0 0 1 1 1
  spline S321 degree 2 poles (1.0734, -0.2256) (1.2205, -0.2256) (1.6017, 0.834) knots 0 0 0 1 1 1
  spline S322 degree 2 poles (1.6017, 0.834) (1.7608, 1.2873) (1.8148, 1.4224) knots 0 0 0 1 1 1
  spline S323 degree 2 poles (1.8148, 1.4224) (1.8748, 1.5394) (1.9979, 1.5394) knots 0 0 0 1 1 1
  spline S324 degree 2 poles (-6.6996, -4.9252) (-6.3304, -4.9252) (-6.0602, -5.1713) knots 0 0 0 1 1 1
  spline S325 degree 2 poles (-6.0602, -5.1713) (-5.7991, -5.4385) (-5.7991, -5.8137) knots 0 0 0 1 1 1
  spline S326 degree 2 poles (-5.7991, -5.8137) (-5.7991, -6.333) (-6.3123, -6.8763) knots 0 0 0 1 1 1
  spline S327 degree 2 poles (-6.3123, -6.8763) (-6.4774, -7.0384) (-6.6005, -7.1374) knots 0 0 0 1 1 1
  spline S328 degree 2 poles (-6.6005, -7.1374) (-6.3033, -7.3175) (-6.1833, -7.6567) knots 0 0 0 1 1 1
  spline S329 degree 2 poles (-6.1833, -7.6567) (-6.1262, -7.8248) (-6.1262, -8.0019) knots 0 0 0 1 1 1
  line L69 (-6.1262, -8.0019) -> (-6.1262, -8.0139)
  spline S330 degree 2 poles (-6.1262, -8.0139) (-6.1262, -8.3471) (-6.3244, -8.6413) knots 0 0 0 1 1 1
  spline S331 degree 2 poles (-6.3244, -8.6413) (-6.5375, -8.9204) (-6.8106, -8.9204) knots 0 0 0 1 1 1
  spline S332 degree 2 poles (-6.8106, -8.9204) (-7.3449, -8.9204) (-7.45, -7.9419) knots 0 0 0 1 1 1
  spline S333 degree 2 poles (-7.45, -7.9419) (-7.474, -7.7168) (-7.474, -7.4526) knots 0 0 0 1 1 1
  spline S334 degree 2 poles (-7.474, -7.4526) (-7.474, -6.8403) (-7.3599, -5.9547) knots 0 0 0 1 1 1
  spline S335 degree 2 poles (-7.3599, -5.9547) (-7.3419, -5.8857) (-7.2759, -5.8347) knots 0 0 0 1 1 1
  spline S336 degree 2 poles (-7.2759, -5.8347) (-7.2159, -5.8077) (-7.1678, -5.8077) knots 0 0 0 1 1 1
  spline S337 degree 2 poles (-7.1678, -5.8077) (-7.0568, -5.8077) (-6.9937, -5.9187) knots 0 0 0 1 1 1
  spline S338 degree 2 poles (-6.9937, -5.9187) (-6.9787, -5.9577) (-6.9787, -5.9998) knots 0 0 0 1 1 1
  line L70 (-6.9787, -5.9998) -> (-6.9787, -6.0028)
  spline S339 degree 2 poles (-6.9787, -6.0028) (-7.0358, -6.459) (-7.0718, -6.9993) knots 0 0 0 1 1 1
  spline S340 degree 2 poles (-7.0718, -6.9993) (-6.9217, -6.9033) (-6.6876, -6.6992) knots 0 0 0 1 1 1
  spline S341 degree 2 poles (-6.6876, -6.6992) (-6.1863, -6.2279) (-6.1863, -5.8167) knots 0 0 0 1 1 1
  line L71 (-6.1863, -5.8167) -> (-6.1863, -5.8107)
  spline S342 degree 2 poles (-6.1863, -5.8107) (-6.1863, -5.5285) (-6.4234, -5.3844) knots 0 0 0 1 1 1
  spline S343 degree 2 poles (-6.4234, -5.3844) (-6.5525, -5.3124) (-6.6725, -5.3124) knots 0 0 0 1 1 1
  line L72 (-6.6725, -5.3124) -> (-6.7296, -5.3124)
  spline S344 degree 2 poles (-6.7296, -5.3124) (-6.9277, -5.3124) (-7.1768, -5.4715) knots 0 0 0 1 1 1
  spline S345 degree 2 poles (-7.1768, -5.4715) (-7.2549, -5.5255) (-7.3389, -5.6065) knots 0 0 0 1 1 1
  spline S346 degree 2 poles (-7.3389, -5.6065) (-7.504, -5.7686) (-7.5521, -5.8467) knots 0 0 0 1 1 1
  spline S347 degree 2 poles (-7.5521, -5.8467) (-7.7352, -6.1138) (-7.8402, -6.387) knots 0 0 0 1 1 1
  spline S348 degree 2 poles (-7.8402, -6.387) (-7.9063, -6.5401) (-7.9753, -6.7772) knots 0 0 0 1 1 1
  spline S349 degree 2 poles (-7.9753, -6.7772) (-8.0353, -6.8943) (-8.1584, -6.8943) knots 0 0 0 1 1 1
  spline S350 degree 2 poles (-8.1584, -6.8943) (-8.2665, -6.8943) (-8.3295, -6.7802) knots 0 0 0 1 1 1
  spline S351 degree 2 poles (-8.3295, -6.7802) (-8.3475, -6.7442) (-8.3475, -6.6992) knots 0 0 0 1 1 1
  spline S352 degree 2 poles (-8.3475, -6.6992) (-8.3355, -6.5491) (-8.1254, -6.0658) knots 0 0 0 1 1 1
  spline S353 degree 2 poles (-8.1254, -6.0658) (-8.0113, -5.8257) (-7.8252, -5.5675) knots 0 0 0 1 1 1
  spline S354 degree 2 poles (-7.8252, -5.5675) (-7.7592, -5.4715) (-7.5611, -5.2824) knots 0 0 0 1 1 1
  spline S355 degree 2 poles (-7.5611, -5.2824) (-7.1498, -4.9252) (-6.6996, -4.9252) knots 0 0 0 1 1 1
  line L73 (-7.0838, -7.3505) -> (-7.0838, -7.4736)
  spline S356 degree 2 poles (-7.0838, -7.4736) (-7.0838, -8.095) (-6.9547, -8.4162) knots 0 0 0 1 1 1
  spline S357 degree 2 poles (-6.9547, -8.4162) (-6.8917, -8.5302) (-6.8316, -8.5302) knots 0 0 0 1 1 1
  line L74 (-6.8316, -8.5302) -> (-6.8076, -8.5302)
  spline S358 degree 2 poles (-6.8076, -8.5302) (-6.6906, -8.5302) (-6.5705, -8.3021) knots 0 0 0 1 1 1
  spline S359 degree 2 poles (-6.5705, -8.3021) (-6.5105, -8.149) (-6.5105, -8.0049) knots 0 0 0 1 1 1
  spline S360 degree 2 poles (-6.5105, -8.0049) (-6.5105, -7.6357) (-6.8587, -7.4406) knots 0 0 0 1 1 1
  spline S361 degree 2 poles (-6.8587, -7.4406) (-6.9547, -7.3926) (-7.0778, -7.3535) knots 0 0 0 1 1 1
  spline S362 degree 2 poles (-7.0778, -7.3535) (-7.0778, -7.3535) (-7.0838, -7.3505) knots 0 0 0 1 1 1
  spline S363 degree 2 poles (-5.2738, -5.3514) (-5.1387, -5.3514) (-5.0876, -5.4985) knots 0 0 0 1 1 1
  spline S364 degree 2 poles (-5.0876, -5.4985) (-5.0816, -5.5225) (-5.0816, -5.5375) knots 0 0 0 1 1 1
  line L75 (-5.0816, -5.5375) -> (-5.0816, -5.5585)
  spline S365 degree 2 poles (-5.0816, -5.5585) (-5.0816, -5.6246) (-5.1537, -5.7086) knots 0 0 0 1 1 1
  spline S366 degree 2 poles (-5.1537, -5.7086) (-5.3548, -6.0718) (-5.3548, -6.7832) knots 0 0 0 1 1 1
  spline S367 degree 2 poles (-5.3548, -6.7832) (-5.3548, -7.5577) (-5.1147, -8.0529) knots 0 0 0 1 1 1
  spline S368 degree 2 poles (-5.1147, -8.0529) (-5.0576, -8.17) (-4.9436, -8.2841) knots 0 0 0 1 1 1
  spline S369 degree 2 poles (-4.9436, -8.2841) (-4.7755, -8.4612) (-4.6464, -8.4612) knots 0 0 0 1 1 1
  line L76 (-4.6464, -8.4612) -> (-4.6374, -8.4612)
  spline S370 degree 2 poles (-4.6374, -8.4612) (-4.4753, -8.4612) (-4.3102, -8.122) knots 0 0 0 1 1 1
  spline S371 degree 2 poles (-4.3102, -8.122) (-4.0701, -7.5607) (-4.0701, -6.8012) knots 0 0 0 1 1 1
  spline S372 degree 2 poles (-4.0701, -6.8012) (-4.0701, -6.2099) (-4.2412, -5.7806) knots 0 0 0 1 1 1
  line L77 (-4.2412, -5.7806) -> (-4.2472, -5.7386)
  spline S373 degree 2 poles (-4.2472, -5.7386) (-4.2472, -5.6216) (-4.1211, -5.5585) knots 0 0 0 1 1 1
  spline S374 degree 2 poles (-4.1211, -5.5585) (-4.0821, -5.5465) (-4.0521, -5.5465) knots 0 0 0 1 1 1
  spline S375 degree 2 poles (-4.0521, -5.5465) (-3.908, -5.5465) (-3.8509, -5.7176) knots 0 0 0 1 1 1
  spline S376 degree 2 poles (-3.8509, -5.7176) (-3.6828, -6.1829) (-3.6828, -6.8162) knots 0 0 0 1 1 1
  spline S377 degree 2 poles (-3.6828, -6.8162) (-3.6828, -7.5637) (-3.908, -8.176) knots 0 0 0 1 1 1
  spline S378 degree 2 poles (-3.908, -8.176) (-3.992, -8.3831) (-4.1121, -8.5482) knots 0 0 0 1 1 1
  spline S379 degree 2 poles (-4.1121, -8.5482) (-4.3492, -8.8484) (-4.6224, -8.8484) knots 0 0 0 1 1 1
  line L78 (-4.6224, -8.8484) -> (-4.6554, -8.8484)
  spline S380 degree 2 poles (-4.6554, -8.8484) (-4.9826, -8.8484) (-5.3278, -8.4402) knots 0 0 0 1 1 1
  spline S381 degree 2 poles (-5.3278, -8.4402) (-5.4088, -8.3231) (-5.4599, -8.233) knots 0 0 0 1 1 1
  spline S382 degree 2 poles (-5.4599, -8.233) (-5.5499, -8.0529) (-5.631, -7.7588) knots 0 0 0 1 1 1
  spline S383 degree 2 poles (-5.631, -7.7588) (-5.745, -7.2965) (-5.745, -6.7982) knots 0 0 0 1 1 1
  spline S384 degree 2 poles (-5.745, -6.7982) (-5.745, -6.1469) (-5.5679, -5.6726) knots 0 0 0 1 1 1
  spline S385 degree 2 poles (-5.5679, -5.6726) (-5.5079, -5.5345) (-5.4298, -5.4294) knots 0 0 0 1 1 1
  spline S386 degree 2 poles (-5.4298, -5.4294) (-5.3698, -5.3514) (-5.2738, -5.3514) knots 0 0 0 1 1 1
  line L79 (-2.6713, -9.0375) -> (-2.6803, -9.0375)
  spline S387 degree 2 poles (-2.6803, -9.0375) (-2.8754, -9.0015) (-2.8754, -8.8454) knots 0 0 0 1 1 1
  spline S388 degree 2 poles (-2.8754, -8.8454) (-2.8274, -8.6623) (-2.8274, -8.092) knots 0 0 0 1 1 1
  spline S389 degree 2 poles (-2.8274, -8.092) (-2.8364, -7.8218) (-2.8364, -7.7498) knots 0 0 0 1 1 1
  spline S390 degree 2 poles (-2.8364, -7.7498) (-2.9954, -7.7498) (-3.0345, -7.5427) knots 0 0 0 1 1 1
  spline S391 degree 2 poles (-3.0345, -7.5427) (-2.9864, -7.3475) (-2.8454, -7.3475) knots 0 0 0 1 1 1
  line L80 (-2.8454, -7.3475) -> (-2.8754, -6.1529)
  spline S392 degree 2 poles (-2.8754, -6.1529) (-2.8754, -5.9307) (-2.6893, -5.9247) knots 0 0 0 1 1 1
  line L81 (-2.6893, -5.9247) -> (-2.6623, -5.9247)
  spline S393 degree 2 poles (-2.6623, -5.9247) (-2.4852, -5.9217) (-2.4762, -6.1228) knots 0 0 0 1 1 1
  spline S394 degree 2 poles (-2.4762, -6.1228) (-2.4852, -6.414) (-2.4461, -7.3776) knots 0 0 0 1 1 1
  spline S395 degree 2 poles (-2.4461, -7.3776) (-2.0049, -7.3776) (-1.7707, -6.9453) knots 0 0 0 1 1 1
  spline S396 degree 2 poles (-1.7707, -6.9453) (-1.6927, -6.7892) (-1.6927, -6.6061) knots 0 0 0 1 1 1
  line L82 (-1.6927, -6.6061) -> (-1.6927, -6.5161)
  spline S397 degree 2 poles (-1.6927, -6.5161) (-1.6927, -6.0928) (-1.9869, -5.7837) knots 0 0 0 1 1 1
  spline S398 degree 2 poles (-1.9869, -5.7837) (-2.188, -5.6276) (-2.4161, -5.6276) knots 0 0 0 1 1 1
  spline S399 degree 2 poles (-2.4161, -5.6276) (-2.7883, -5.6276) (-2.9564, -5.9397) knots 0 0 0 1 1 1
  spline S400 degree 2 poles (-2.9564, -5.9397) (-3.0105, -6.1439) (-3.1515, -6.1439) knots 0 0 0 1 1 1
  line L83 (-3.1515, -6.1439) -> (-3.1996, -6.1439)
  spline S401 degree 2 poles (-3.1996, -6.1439) (-3.3316, -6.1439) (-3.3647, -5.9487) knots 0 0 0 1 1 1
  spline S402 degree 2 poles (-3.3647, -5.9487) (-3.3647, -5.7326) (-3.0615, -5.4505) knots 0 0 0 1 1 1
  spline S403 degree 2 poles (-3.0615, -5.4505) (-2.7763, -5.2343) (-2.4161, -5.2343) knots 0 0 0 1 1 1
  spline S404 degree 2 poles (-2.4161, -5.2343) (-1.6117, -5.2343) (-1.3385, -6.1649) knots 0 0 0 1 1 1
  spline S405 degree 2 poles (-1.3385, -6.1649) (-1.2905, -6.408) (-1.2905, -6.5761) knots 0 0 0 1 1 1
  spline S406 degree 2 poles (-1.2905, -6.5761) (-1.2905, -7.3355) (-2.0139, -7.6897) knots 0 0 0 1 1 1
  spline S407 degree 2 poles (-2.0139, -7.6897) (-2.152, -7.7288) (-2.173, -7.7288) knots 0 0 0 1 1 1
  spline S408 degree 2 poles (-2.173, -7.7288) (-1.9749, -8.0559) (-1.7527, -8.2961) knots 0 0 0 1 1 1
  spline S409 degree 2 poles (-1.7527, -8.2961) (-1.6567, -8.3921) (-1.5966, -8.4041) knots 0 0 0 1 1 1
  spline S410 degree 2 poles (-1.5966, -8.4041) (-1.4916, -8.2751) (-1.4195, -8.2751) knots 0 0 0 1 1 1
  line L84 (-1.4195, -8.2751) -> (-1.3805, -8.2751)
  spline S411 degree 2 poles (-1.3805, -8.2751) (-1.2304, -8.2751) (-1.1944, -8.4732) knots 0 0 0 1 1 1
  spline S412 degree 2 poles (-1.1944, -8.4732) (-1.1944, -8.6533) (-1.5066, -8.7854) knots 0 0 0 1 1 1
  spline S413 degree 2 poles (-1.5066, -8.7854) (-1.5456, -8.7944) (-1.5876, -8.7944) knots 0 0 0 1 1 1
  spline S414 degree 2 poles (-1.5876, -8.7944) (-1.9629, -8.7944) (-2.4071, -8.092) knots 0 0 0 1 1 1
  line L85 (-2.4071, -8.092) -> (-2.4371, -8.062)
  line L86 (-2.4371, -8.062) -> (-2.4371, -8.227)
  spline S415 degree 2 poles (-2.4371, -8.227) (-2.4371, -8.9715) (-2.5332, -8.9715) knots 0 0 0 1 1 1
  spline S416 degree 2 poles (-2.5332, -8.9715) (-2.5332, -9.0135) (-2.6713, -9.0375) knots 0 0 0 1 1 1
  line L87 (0.9188, -5.3994) -> (0.9518, -5.3994)
  spline S417 degree 2 poles (0.9518, -5.3994) (1.0299, -5.3994) (1.1019, -5.4925) knots 0 0 0 1 1 1
  spline S418 degree 2 poles (1.1019, -5.4925) (1.1349, -5.5345) (1.1349, -5.7236) knots 0 0 0 1 1 1
  spline S419 degree 2 poles (1.1349, -5.7236) (1.1589, -6.381) (1.1589, -6.9333) knots 0 0 0 1 1 1
  line L88 (1.1589, -6.9333) -> (1.1589, -6.9603)
  spline S420 degree 2 poles (1.1589, -6.9603) (1.1589, -8.215) (0.9908, -8.5302) knots 0 0 0 1 1 1
  spline S421 degree 2 poles (0.9908, -8.5302) (0.9248, -8.6473) (0.8287, -8.6473) knots 0 0 0 1 1 1
  spline S422 degree 2 poles (0.8287, -8.6473) (0.6216, -8.6473) (0.4025, -8.164) knots 0 0 0 1 1 1
  spline S423 degree 2 poles (0.4025, -8.164) (0.2884, -7.9149) (0.0063, -7.2245) knots 0 0 0 1 1 1
  spline S424 degree 2 poles (0.0063, -7.2245) (-0.2399, -6.6541) (-0.471, -6.2939) knots 0 0 0 1 1 1
  line L89 (-0.471, -6.2939) -> (-0.474, -6.2939)
  spline S425 degree 2 poles (-0.474, -6.2939) (-0.474, -6.342) (-0.477, -6.5161) knots 0 0 0 1 1 1
  line L90 (-0.477, -6.5161) -> (-0.468, -7.7047)
  spline S426 degree 2 poles (-0.468, -7.7047) (-0.468, -8.7614) (-0.6151, -8.8484) knots 0 0 0 1 1 1
  spline S427 degree 2 poles (-0.6151, -8.8484) (-0.6691, -8.8964) (-0.7292, -8.8964) knots 0 0 0 1 1 1
  line L91 (-0.7292, -8.8964) -> (-0.7382, -8.8964)
  spline S428 degree 2 poles (-0.7382, -8.8964) (-0.8702, -8.8964) (-0.9243, -8.7553) knots 0 0 0 1 1 1
  spline S429 degree 2 poles (-0.9243, -8.7553) (-0.9333, -8.7223) (-0.9333, -8.7013) knots 0 0 0 1 1 1
  spline S430 degree 2 poles (-0.9333, -8.7013) (-0.9333, -8.6803) (-0.9003, -8.5452) knots 0 0 0 1 1 1
  spline S431 degree 2 poles (-0.9003, -8.5452) (-0.8552, -8.3021) (-0.8552, -7.7738) knots 0 0 0 1 1 1
  line L92 (-0.8552, -7.7738) -> (-0.8552, -7.6927)
  spline S432 degree 2 poles (-0.8552, -7.6927) (-0.8552, -7.4706) (-0.8642, -6.7592) knots 0 0 0 1 1 1
  spline S433 degree 2 poles (-0.8642, -6.7592) (-0.8642, -5.9157) (-0.7262, -5.7867) knots 0 0 0 1 1 1
  spline S434 degree 2 poles (-0.7262, -5.7867) (-0.6361, -5.7026) (-0.5581, -5.7026) knots 0 0 0 1 1 1
  spline S435 degree 2 poles (-0.5581, -5.7026) (-0.417, -5.7026) (-0.2339, -5.9577) knots 0 0 0 1 1 1
  spline S436 degree 2 poles (-0.2339, -5.9577) (-0.0538, -6.2039) (0.1233, -6.5551) knots 0 0 0 1 1 1
  spline S437 degree 2 poles (0.1233, -6.5551) (0.3605, -7.0414) (0.7057, -7.8969) knots 0 0 0 1 1 1
  spline S438 degree 2 poles (0.7057, -7.8969) (0.7567, -8.0169) (0.7807, -8.0379) knots 0 0 0 1 1 1
  line L93 (0.7807, -8.0379) -> (0.7897, -8.0379)
  spline S439 degree 2 poles (0.7897, -8.0379) (0.7987, -7.9209) (0.7987, -7.7528) knots 0 0 0 1 1 1
  spline S440 degree 2 poles (0.7987, -7.7528) (0.7987, -7.1464) (0.7417, -5.5885) knots 0 0 0 1 1 1
  spline S441 degree 2 poles (0.7417, -5.5885) (0.7417, -5.4895) (0.8497, -5.4204) knots 0 0 0 1 1 1
  spline S442 degree 2 poles (0.8497, -5.4204) (0.8948, -5.3994) (0.9188, -5.3994) knots 0 0 0 1 1 1
  line L94 (2.1705, -5.2914) -> (2.1975, -5.2914)
  spline S443 degree 2 poles (2.1975, -5.2914) (2.2966, -5.2914) (2.3626, -5.4054) knots 0 0 0 1 1 1
  spline S444 degree 2 poles (2.3626, -5.4054) (2.3716, -5.4324) (2.3716, -5.4355) knots 0 0 0 1 1 1
  spline S445 degree 2 poles (2.3716, -5.4355) (2.6508, -5.4264) (2.6508, -5.4084) knots 0 0 0 1 1 1